Autodesk Fusion 360 part; units mm, degrees
(part 2 of 2)
sketch "Esboço7 (7)" plane through (0, 0, 0) normal (0, 0, 1) x (1, 0, 0) in component "SmartMeter_VentilationGrille"
  line L0 (-34, 10.75) -> (34, 10.75)
  line L1 (34, 10.75) -> (34, 14.25)
  line L2 (34, 14.25) -> (-34, 14.25)
  line L3 (-34, 14.25) -> (-34, 10.75)
extrude "07_cut_rect (1)'" cut sketch "Esboço7 (7)" along normal blind 3.5 bodies 30 in component "SmartMeter_VentilationGrille"
sketch "Esboço8 (6)" plane through (0, 0, 0) normal (0, 0, 1) x (1, 0, 0) in component "SmartMeter_VentilationGrille"
  circle A0 centre (-39, -12) radius 1.6
extrude "08_cut_circle (1)'''" cut sketch "Esboço8 (6)" along normal blind 3.5 bodies 30 in component "SmartMeter_VentilationGrille"
sketch "Esboço9 (6)" plane through (0, 0, 0) normal (0, 0, 1) x (1, 0, 0) in component "SmartMeter_VentilationGrille"
  circle A0 centre (-39, 12) radius 1.6
extrude "09_cut_circle (1)'''" cut sketch "Esboço9 (6)" along normal blind 3.5 bodies 30 in component "SmartMeter_VentilationGrille"
sketch "Esboço10 (6)" plane through (0, 0, 0) normal (0, 0, 1) x (1, 0, 0) in component "SmartMeter_VentilationGrille"
  circle A0 centre (39, -12) radius 1.6
extrude "10_cut_circle (1)''''" cut sketch "Esboço10 (6)" along normal blind 3.5 bodies 30 in component "SmartMeter_VentilationGrille"
sketch "Esboço11 (5)" plane through (0, 0, 0) normal (0, 0, 1) x (1, 0, 0) in component "SmartMeter_VentilationGrille"
  circle A0 centre (39, 12) radius 1.6
extrude "11_cut_circle (1)''" cut sketch "Esboço11 (5)" along normal blind 3.5 bodies 30 in component "SmartMeter_VentilationGrille"
sketch "Esboço1 (9)" plane through (0, 0, 0) normal (0, 0, 1) x (1, 0, 0) in component "SmartMeter_MetrologyCarrier"
  line L0 (-42.5, -47.5) -> (42.5, -47.5)
  line L1 (42.5, -47.5) -> (42.5, 47.5)
  line L2 (42.5, 47.5) -> (-42.5, 47.5)
  line L3 (-42.5, 47.5) -> (-42.5, -47.5)
extrude "01_new_rect (1)'''''''" add sketch "Esboço1 (9)" along normal blind 3 separate body makes body 31 in component "SmartMeter_MetrologyCarrier"
sketch "Esboço2 (9)" plane through (0, 0, 0) normal (0, 0, 1) x (1, 0, 0) in component "SmartMeter_MetrologyCarrier"
  circle A0 centre (-32.5, -37.5) radius 1.6
extrude "02_cut_circle (1)'" cut sketch "Esboço2 (9)" along normal blind 3 bodies 31 in component "SmartMeter_MetrologyCarrier"
sketch "Esboço3 (9)" plane through (0, 0, 0) normal (0, 0, 1) x (1, 0, 0) in component "SmartMeter_MetrologyCarrier"
  circle A0 centre (-32.5, 37.5) radius 1.6
extrude "03_cut_circle (1)'''" cut sketch "Esboço3 (9)" along normal blind 3 bodies 31 in component "SmartMeter_MetrologyCarrier"
sketch "Esboço4 (9)" plane through (0, 0, 0) normal (0, 0, 1) x (1, 0, 0) in component "SmartMeter_MetrologyCarrier"
  circle A0 centre (32.5, -37.5) radius 1.6
extrude "04_cut_circle (1)''''" cut sketch "Esboço4 (9)" along normal blind 3 bodies 31 in component "SmartMeter_MetrologyCarrier"
sketch "Esboço5 (9)" plane through (0, 0, 0) normal (0, 0, 1) x (1, 0, 0) in component "SmartMeter_MetrologyCarrier"
  circle A0 centre (32.5, 37.5) radius 1.6
extrude "05_cut_circle (1)'''''" cut sketch "Esboço5 (9)" along normal blind 3 bodies 31 in component "SmartMeter_MetrologyCarrier"
sketch "Esboço6 (9)" plane through (0, 0, 0) normal (0, 0, 1) x (1, 0, 0) in component "SmartMeter_MetrologyCarrier"
  circle A0 centre (-30, -30) radius 1.6
extrude "06_cut_circle (1)'''''" cut sketch "Esboço6 (9)" along normal blind 3 bodies 31 in component "SmartMeter_MetrologyCarrier"
sketch "Esboço7 (8)" plane through (0, 0, 0) normal (0, 0, 1) x (1, 0, 0) in component "SmartMeter_MetrologyCarrier"
  circle A0 centre (-30, 30) radius 1.6
extrude "07_cut_circle (1)''''" cut sketch "Esboço7 (8)" along normal blind 3 bodies 31 in component "SmartMeter_MetrologyCarrier"
sketch "Esboço8 (7)" plane through (0, 0, 0) normal (0, 0, 1) x (1, 0, 0) in component "SmartMeter_MetrologyCarrier"
  circle A0 centre (30, -30) radius 1.6
extrude "08_cut_circle (1)''''" cut sketch "Esboço8 (7)" along normal blind 3 bodies 31 in component "SmartMeter_MetrologyCarrier"
sketch "Esboço9 (7)" plane through (0, 0, 0) normal (0, 0, 1) x (1, 0, 0) in component "SmartMeter_MetrologyCarrier"
  circle A0 centre (30, 30) radius 1.6
extrude "09_cut_circle (1)''''" cut sketch "Esboço9 (7)" along normal blind 3 bodies 31 in component "SmartMeter_MetrologyCarrier"
sketch "Esboço1 (10)" plane through (0, 0, 0) normal (0, 0, 1) x (1, 0, 0) in component "SmartMeter_HmiCarrier"
  line L0 (-52.5, -37.5) -> (52.5, -37.5)
  line L1 (52.5, -37.5) -> (52.5, 37.5)
  line L2 (52.5, 37.5) -> (-52.5, 37.5)
  line L3 (-52.5, 37.5) -> (-52.5, -37.5)
extrude "01_new_rect (1)''''''''" add sketch "Esboço1 (10)" along normal blind 3 separate body makes body 32 in component "SmartMeter_HmiCarrier"
sketch "Esboço2 (10)" plane through (0, 0, 0) normal (0, 0, 1) x (1, 0, 0) in component "SmartMeter_HmiCarrier"
  circle A0 centre (-42.5, -27.5) radius 1.6
extrude "02_cut_circle (1)''" cut sketch "Esboço2 (10)" along normal blind 3 bodies 32 in component "SmartMeter_HmiCarrier"
sketch "Esboço3 (10)" plane through (0, 0, 0) normal (0, 0, 1) x (1, 0, 0) in component "SmartMeter_HmiCarrier"
  circle A0 centre (-42.5, 27.5) radius 1.6
extrude "03_cut_circle (1)''''" cut sketch "Esboço3 (10)" along normal blind 3 bodies 32 in component "SmartMeter_HmiCarrier"
sketch "Esboço4 (10)" plane through (0, 0, 0) normal (0, 0, 1) x (1, 0, 0) in component "SmartMeter_HmiCarrier"
  circle A0 centre (42.5, -27.5) radius 1.6
extrude "04_cut_circle (1)'''''" cut sketch "Esboço4 (10)" along normal blind 3 bodies 32 in component "SmartMeter_HmiCarrier"
sketch "Esboço5 (10)" plane through (0, 0, 0) normal (0, 0, 1) x (1, 0, 0) in component "SmartMeter_HmiCarrier"
  circle A0 centre (42.5, 27.5) radius 1.6
extrude "05_cut_circle (1)''''''" cut sketch "Esboço5 (10)" along normal blind 3 bodies 32 in component "SmartMeter_HmiCarrier"
sketch "Esboço6 (10)" plane through (0, 0, 0) normal (0, 0, 1) x (1, 0, 0) in component "SmartMeter_HmiCarrier"
  circle A0 centre (-35, -25) radius 1.6
extrude "06_cut_circle (1)''''''" cut sketch "Esboço6 (10)" along normal blind 3 bodies 32 in component "SmartMeter_HmiCarrier"
sketch "Esboço7 (9)" plane through (0, 0, 0) normal (0, 0, 1) x (1, 0, 0) in component "SmartMeter_HmiCarrier"
  circle A0 centre (-35, 25) radius 1.6
extrude "07_cut_circle (1)'''''" cut sketch "Esboço7 (9)" along normal blind 3 bodies 32 in component "SmartMeter_HmiCarrier"
sketch "Esboço8 (8)" plane through (0, 0, 0) normal (0, 0, 1) x (1, 0, 0) in component "SmartMeter_HmiCarrier"
  circle A0 centre (35, -25) radius 1.6
extrude "08_cut_circle (1)'''''" cut sketch "Esboço8 (8)" along normal blind 3 bodies 32 in component "SmartMeter_HmiCarrier"
sketch "Esboço9 (8)" plane through (0, 0, 0) normal (0, 0, 1) x (1, 0, 0) in component "SmartMeter_HmiCarrier"
  circle A0 centre (35, 25) radius 1.6
extrude "09_cut_circle (1)'''''" cut sketch "Esboço9 (8)" along normal blind 3 bodies 32 in component "SmartMeter_HmiCarrier"
sketch "Esboço10 (7)" plane through (0, 0, 0) normal (0, 0, 1) x (1, 0, 0) in component "SmartMeter_HmiCarrier"
  circle A0 centre (-27.5, -17.5) radius 5
extrude "Extrusão10'" add sketch "Esboço10 (7)" along normal blind 12 separate body makes body 33 in component "SmartMeter_HmiCarrier"
combine "10_join_circle (1)'" operation add target body 32 tool bodies 33 in component "SmartMeter_HmiCarrier"
sketch "Esboço11 (6)" plane through (0, 0, 0) normal (0, 0, 1) x (1, 0, 0) in component "SmartMeter_HmiCarrier"
  circle A0 centre (-27.5, 17.5) radius 5
extrude "Extrusão11" add sketch "Esboço11 (6)" along normal blind 12 separate body makes body 34 in component "SmartMeter_HmiCarrier"
combine "11_join_circle (1)" operation add target body 32 tool bodies 34 in component "SmartMeter_HmiCarrier"
sketch "Esboço12 (4)" plane through (0, 0, 0) normal (0, 0, 1) x (1, 0, 0) in component "SmartMeter_HmiCarrier"
  circle A0 centre (27.5, -17.5) radius 5
extrude "Extrusão12" add sketch "Esboço12 (4)" along normal blind 12 separate body makes body 35 in component "SmartMeter_HmiCarrier"
combine "12_join_circle (1)" operation add target body 32 tool bodies 35 in component "SmartMeter_HmiCarrier"
sketch "Esboço13 (4)" plane through (0, 0, 0) normal (0, 0, 1) x (1, 0, 0) in component "SmartMeter_HmiCarrier"
  circle A0 centre (27.5, 17.5) radius 5
extrude "Extrusão13" add sketch "Esboço13 (4)" along normal blind 12 separate body makes body 36 in component "SmartMeter_HmiCarrier"
combine "13_join_circle (1)" operation add target body 32 tool bodies 36 in component "SmartMeter_HmiCarrier"
ref_plane "Plano de trabalho1" through (0, 0, 3) normal (0, 0, 1) x (1, 0, 0) in component "SmartMeter_HmiCarrier"
sketch "Esboço14 (3)" plane through (0, 0, 3) normal (0, 0, 1) x (1, 0, 0) in component "SmartMeter_HmiCarrier"
  circle A0 centre (-27.5, -17.5) radius 1.6
extrude "14_cut_circle (1)''" cut sketch "Esboço14 (3)" along normal blind 9 bodies 32 in component "SmartMeter_HmiCarrier"
ref_plane "Plano de trabalho2" through (0, 0, 3) normal (0, 0, 1) x (1, 0, 0) in component "SmartMeter_HmiCarrier"
sketch "Esboço15 (3)" plane through (0, 0, 3) normal (0, 0, 1) x (1, 0, 0) in component "SmartMeter_HmiCarrier"
  circle A0 centre (-27.5, 17.5) radius 1.6
extrude "15_cut_circle (1)''" cut sketch "Esboço15 (3)" along normal blind 9 bodies 32 in component "SmartMeter_HmiCarrier"
ref_plane "Plano de trabalho3" through (0, 0, 3) normal (0, 0, 1) x (1, 0, 0) in component "SmartMeter_HmiCarrier"
sketch "Esboço16 (3)" plane through (0, 0, 3) normal (0, 0, 1) x (1, 0, 0) in component "SmartMeter_HmiCarrier"
  circle A0 centre (27.5, -17.5) radius 1.6
extrude "16_cut_circle (1)'" cut sketch "Esboço16 (3)" along normal blind 9 bodies 32 in component "SmartMeter_HmiCarrier"
ref_plane "Plano de trabalho4" through (0, 0, 3) normal (0, 0, 1) x (1, 0, 0) in component "SmartMeter_HmiCarrier"
sketch "Esboço17 (3)" plane through (0, 0, 3) normal (0, 0, 1) x (1, 0, 0) in component "SmartMeter_HmiCarrier"
  circle A0 centre (27.5, 17.5) radius 1.6
extrude "17_cut_circle (1)'" cut sketch "Esboço17 (3)" along normal blind 9 bodies 32 in component "SmartMeter_HmiCarrier"
sketch "Esboço1 (11)" plane through (0, 0, 0) normal (0, 0, 1) x (1, 0, 0) in component "SmartMeter_CommCarrier"
  line L0 (-37.5, -27.5) -> (37.5, -27.5)
  line L1 (37.5, -27.5) -> (37.5, 27.5)
  line L2 (37.5, 27.5) -> (-37.5, 27.5)
  line L3 (-37.5, 27.5) -> (-37.5, -27.5)
extrude "01_new_rect (1)'''''''''" add sketch "Esboço1 (11)" along normal blind 3 separate body makes body 37 in component "SmartMeter_CommCarrier"
sketch "Esboço2 (11)" plane through (0, 0, 0) normal (0, 0, 1) x (1, 0, 0) in component "SmartMeter_CommCarrier"
  circle A0 centre (-27.5, -17.5) radius 1.6
extrude "02_cut_circle (1)'''" cut sketch "Esboço2 (11)" along normal blind 3 bodies 37 in component "SmartMeter_CommCarrier"
sketch "Esboço3 (11)" plane through (0, 0, 0) normal (0, 0, 1) x (1, 0, 0) in component "SmartMeter_CommCarrier"
  circle A0 centre (-27.5, 17.5) radius 1.6
extrude "03_cut_circle (1)'''''" cut sketch "Esboço3 (11)" along normal blind 3 bodies 37 in component "SmartMeter_CommCarrier"
sketch "Esboço4 (11)" plane through (0, 0, 0) normal (0, 0, 1) x (1, 0, 0) in component "SmartMeter_CommCarrier"
  circle A0 centre (27.5, -17.5) radius 1.6
extrude "04_cut_circle (1)''''''" cut sketch "Esboço4 (11)" along normal blind 3 bodies 37 in component "SmartMeter_CommCarrier"
sketch "Esboço5 (11)" plane through (0, 0, 0) normal (0, 0, 1) x (1, 0, 0) in component "SmartMeter_CommCarrier"
  circle A0 centre (27.5, 17.5) radius 1.6
extrude "05_cut_circle (1)'''''''" cut sketch "Esboço5 (11)" along normal blind 3 bodies 37 in component "SmartMeter_CommCarrier"
component "SmartMeter_DesktopFeet" placed x (1, 0, 0) y (0, 0, 1) z (0, -1, 0) at (0, -72.5, 40)
component "SmartMeter_DisplayBracket" placed x (1, 0, 0) y (0, 1, 0) z (0, 0, 1) at (0, 0, 0)
component "SmartMeter_FrontPanel" placed x (1, 0, 0) y (0, 1, 0) z (0, 0, 1) at (0, 0, -4)
component "SmartMeter_InternalTray" placed x (1, 0, 0) y (0, 1, 0) z (0, 0, 1) at (0, 0, 40)
component "SmartMeter_PanelMountFrame" placed x (1, 0, 0) y (0, 1, 0) z (0, 0, 1) at (0, 0, -8)
component "SmartMeter_RearHousing" placed x (1, 0, 0) y (0, 1, 0) z (0, 0, 1) at (0, 0, 0)
component "SmartMeter_RearPanel" placed x (1, 0, 0) y (0, 1, 0) z (0, 0, 1) at (0, 0, 75)
component "SmartMeter_VentilationGrille" placed x (1, 0, 0) y (0, 0, -1) z (0, 1, 0) at (45, 72.5, 40)
component "SmartMeter_MetrologyCarrier" placed x (1, 0, 0) y (0, 1, 0) z (0, 0, 1) at (-56, 0, 51)
component "SmartMeter_HmiCarrier" placed x (1, 0, 0) y (0, 1, 0) z (0, 0, 1) at (45, 0, 51)
component "SmartMeter_CommCarrier" placed x (1, 0, 0) y (0, 1, 0) z (0, 0, 1) at (45, 0, 63)
